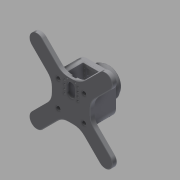
# Autodesk Inventor part: Arm - mounting v2
Saved by Autodesk Inventor 2017 (Build 210142000, 142)
## iProperties
Created: 2017-04-12
Part Number: Arm - mounting v2
Material: Generic
Document SubType Name: Modeling
Designer: Ali
Density: 1 g/cm^3
Appearance: Default
Author: Ali
Autodesk Inventor part; units mm, degrees
ref_plane "YZ Plane" through (0, 0, 0) normal (1, 0, 0) x (0, 1, 0)
ref_plane "XZ Plane" through (0, 0, 0) normal (0, 1, 0) x (-1, 0, 0)
ref_plane "XY Plane" through (0, 0, 0) normal (0, 0, 1) x (1, 0, 0)
sketch "Sketch1" plane through (0, 0, 0) normal (0, 1, 0) x (-1, 0, 0)
  line L0 (16.5, -22) -> (-16.5, -22) construction
  line L1 (-16.5, -22) -> (-16.5, 30.8666) construction
  line L2 (-16.5, 39) -> (16.5, 39)
  line L3 (16.5, 39) -> (16.5, 30.8666)
  line L4 (10.5, -16) -> (-10.5, -16) construction
  line L5 (-10.5, -16) -> (-10.5, 6.3097) construction
  line L6 (-10.5, 33) -> (10.5, 33)
  line L7 (10.5, 33) -> (10.5, 6.3097)
  arc A0 (-10.5, 6.3097) -> (10.5, 6.3097) centre (0, 0) ccw
  line L8 (0, 0) -> (0, -19.3758) construction
  arc A1 (16.5, 30.8666) -> (-16.5, 30.8666) centre (0, 0) ccw construction
  line L9 (16.5, 30.8666) -> (16.5, -22) construction
  line L10 (-16.5, 30.8666) -> (-16.5, 39)
  arc A2 (-16.5, 30.8666) -> (16.5, 30.8666) centre (0, 0) ccw
  line L11 (10.5, 6.3097) -> (10.5, -16) construction
  line L12 (-10.5, 6.3097) -> (-10.5, 33)
  arc A3 (10.5, 6.3097) -> (-10.5, 6.3097) centre (0, 0) ccw construction
  point P0 (0, -16)
  point P1 (0, -22)
  dimension "d0" = 21
  dimension "d1" = 24.5
  dimension "d2" = 6
  dimension "d3" = 33
  dimension "d4" = 6
  dimension "d5" = 16
  dimension "d6" = 6
  dimension "d7" = 70
  constraints: 26 end point, 10 parallel, 8 point on circle, 4 centre point, 4 perpendicular, 2 coincident, 2 horizontal, 2 midpoint, 2 point on line, 1 vertical
  measures "d0" distance of L6.start L6.end
  measures "d1" diameter of A0
  measures "d2" distance between parallel lines of L1 L5
  measures "d3" distance from line of point (0, 0) L6
  measures "d4" distance between parallel lines of L2 L6
  measures "d5" distance from line of point (0, 0) L4
  measures "d6" distance between parallel lines of L4 L0
  measures "d7" diameter of A1
extrude "Extrusion1" add sketch "Sketch1" along normal blind 3.5
sketch "Sketch2" plane through (0, 3.5, 0) normal (0, 1, 0) x (1, 0, 0)
  arc A0 (16.5, -30.8666) -> (-16.5, -30.8666) centre (0, 0) ccw projected
  line L0 (16.5, -39) -> (16.5, -30.8666) projected
  line L1 (-16.5, -39) -> (16.5, -39) projected
  line L2 (-16.5, -30.8666) -> (-16.5, -39) projected
  circle A1 centre (0, 0) radius 21
  dimension "d10" = 42
  constraints: 1 centre point, 1 coincident
  measures "d10" diameter of A1
extrude "Extrusion2" add sketch "Sketch2" along normal blind 8
sketch "Sketch3" plane through (0, 0, 0) normal (0, -1, 0) x (1, 0, 0)
  line L0 (-39, -39) -> (39, -39)
  line L1 (39, -39) -> (39, 39)
  line L2 (39, 39) -> (16.5, 39)
  line L3 (-39, 39) -> (-39, -39)
  line L4 (-39, -39) -> (39, 39) construction
  line L5 (39, -39) -> (-39, 39) construction
  line L6 (16.5, 39) -> (-16.5, 39) projected
  arc A0 (-16.5, 30.8666) -> (16.5, 30.8666) centre (0, 0) ccw projected
  line L7 (-16.5, 39) -> (-16.5, 30.8666) projected
  line L8 (-16.5, 39) -> (-39, 39)
  line L9 (16.5, 30.8666) -> (16.5, 39) projected
  line L10 (16.5, 39) -> (-16.5, 39)
  constraints: 18 end point, 4 parallel, 3 collinear, 2 midpoint, 2 perpendicular, 1 horizontal
extrude "Extrusion3" add sketch "Sketch3" against normal blind 8 contours L3 L8 L7 A0 L9 L2 L1 L0
sketch "Sketch4" plane through (0, 0, 0) normal (0, -1, 0) x (1, 0, 0)
  line L0 (-10.5, 6.3097) -> (-10.5, 33) projected
  line L1 (-10.5, 33) -> (10.5, 33) projected
  line L2 (10.5, 33) -> (10.5, 6.3097) projected
  arc A0 (10.5, 6.3097) -> (-10.5, 6.3097) centre (0, 0) ccw projected
  line L3 (-39, 39) -> (-39, -39) projected
  line L4 (-39, -39) -> (39, -39) projected
  line L5 (39, -39) -> (39, 39) projected
  line L6 (16, 39) -> (16, -12)
  line L7 (16, -12) -> (-16, -12)
  line L8 (-16, -12) -> (-16, 39)
  line L9 (0, 0) -> (0, 9.4966) construction
  line L10 (-16, 39) -> (-39, 39)
  line L11 (16, 39) -> (39, 39)
  point P0 (0, -12)
  dimension "d15" = 32
  dimension "d16" = 12
  constraints: 12 end point, 3 perpendicular, 1 centre point, 1 horizontal, 1 midpoint, 1 point on line, 1 vertical
  measures "d15" distance between parallel lines of L8 L6
  measures "d16" distance from line of point (0, 0) L7
extrude "Extrusion4" add sketch "Sketch4" along normal blind 32 contours L10 L8 L7 L6 L11 L5 L4 L3
fillet "Fillet1" radius 19.25 4 edges at (-39, -12, 39) (39, -12, 39) (39, -12, -39) (-39, -12, -39)
sketch "Sketch5" plane through (0, 8, 0) normal (0, 1, 0) x (1, 0, 0)
  arc A0 (-19.75, 39) -> (-39, 19.75) centre (-19.75, 19.75) ccw projected
  line L0 (-39, 19.75) -> (-39, -19.75) projected
  arc A1 (-39, -19.75) -> (-19.75, -39) centre (-19.75, -19.75) ccw projected
  line L1 (-19.75, -39) -> (-16.5, -39) projected
  line L2 (-16.5, -30.8666) -> (-16.5, -39) projected
  arc A2 (16.5, -30.8666) -> (-16.5, -30.8666) centre (0, 0) ccw projected
  line L3 (16.5, -39) -> (16.5, -30.8666) projected
  line L4 (16.5, -39) -> (19.75, -39) projected
  arc A3 (19.75, -39) -> (39, -19.75) centre (19.75, -19.75) ccw projected
  line L5 (39, -19.75) -> (39, 19.75) projected
  arc A4 (39, 19.75) -> (19.75, 39) centre (19.75, 19.75) ccw projected
  line L6 (19.75, 39) -> (-19.75, 39) projected
extrude "Extrusion5" add sketch "Sketch5" along normal up to surface (3.5 mm away)
sketch "Sketch6" plane through (0, -32, 0) normal (0, -1, 0) x (1, 0, 0)
  line L0 (-68.9878, -68.9878) -> (68.9878, 68.9878) construction
  line L1 (-58.3812, -79.5944) -> (-17.7868, -39)
  line L2 (58.3812, 79.5944) -> (17.7868, 39)
  arc A0 (-79.5944, -58.3812) -> (-58.3812, -79.5944) centre (-68.9878, -68.9878) ccw
  arc A1 (79.5944, 58.3812) -> (58.3812, 79.5944) centre (68.9878, 68.9878) ccw
  line L3 (0, 0) -> (195.1269, 0) construction
  line L4 (-68.9878, 68.9878) -> (68.9878, -68.9878) construction
  line L5 (-79.5944, 58.3812) -> (-39, 17.7868)
  line L6 (79.5944, -58.3812) -> (39, -17.7868)
  arc A2 (-58.3812, 79.5944) -> (-79.5944, 58.3812) centre (-68.9878, 68.9878) ccw
  arc A3 (58.3812, -79.5944) -> (79.5944, -58.3812) centre (68.9878, -68.9878) ccw
  line L7 (0, 0) -> (195.1269, 0) construction
  line L8 (-39, 39) -> (-17.7868, 39) construction
  line L9 (39, 39) -> (39, 17.7868) construction
  line L10 (39, -39) -> (17.7868, -39) construction
  line L11 (-39, -39) -> (-39, -17.7868) construction
  line L12 (-39, 39) -> (39, -39) construction
  line L13 (39, 39) -> (-39, -39) construction
  line L14 (39, -19.75) -> (39, 19.75) projected
  line L15 (-39, 17.7868) -> (17.7868, -39) construction
  line L16 (-17.7868, 39) -> (-58.3812, 79.5944)
  line L17 (17.7868, 39) -> (-39, -17.7868) construction
  line L18 (39, 17.7868) -> (79.5944, 58.3812)
  line L19 (39, -17.7868) -> (-17.7868, 39) construction
  line L20 (17.7868, -39) -> (58.3812, -79.5944)
  line L21 (-17.7868, -39) -> (39, 17.7868) construction
  line L22 (-39, -17.7868) -> (-79.5944, -58.3812)
  line L23 (-17.7868, -39) -> (-39, -39) construction
  line L24 (-39, -17.7868) -> (-39, 17.7868)
  line L25 (-39, 17.7868) -> (-39, 39) construction
  line L26 (-17.7868, 39) -> (17.7868, 39)
  line L27 (17.7868, 39) -> (39, 39) construction
  line L28 (39, 17.7868) -> (39, -17.7868)
  line L29 (39, -17.7868) -> (39, -39) construction
  line L30 (17.7868, -39) -> (-17.7868, -39)
  dimension "d22" = 45
  dimension "d23" = 30
  dimension "d24" = 45
  dimension "d25" = 30
  constraints: 64 end point, 36 parallel, 24 tangent, 9 perpendicular, 8 point on circle, 5 horizontal, 5 point on line, 4 centre point, 4 midpoint, 3 collinear, 3 equal length
  measures "d22" angle of L3 L0
  measures "d23" diameter of A1
  measures "d24" angle of L4 L7
  measures "d25" diameter of A3
extrude "Extrusion6" add sketch "Sketch6" along normal blind 8 separate body
fillet "Fillet2" radius 30 8 edges at (39, -36, 17.7868) (39, -36, -17.7868) (17.7868, -36, -39) (-17.7868, -36, -39) (-39, -36, -17.7868) (-39, -36, 17.7868) (-17.7868, -36, 39) (17.7868, -36, 39)
sketch "Sketch7" plane through (0, -32, 0) normal (0, 1, 0) x (1, 0, 0)
  line L0 (-10, -33) -> (10, -33)
  line L1 (-10, 6) -> (10, 6)
  line L2 (-10, -33) -> (-10, 6)
  line L3 (10, -33) -> (10, 6)
  line L4 (0, 0) -> (0, 4.84) construction
  line L5 (-4.5, -33) -> (4.5, -33)
  line L6 (4.5, -33) -> (4.5, -49)
  line L7 (4.5, -49) -> (-4.5, -49)
  line L8 (-4.5, -49) -> (-4.5, -33)
  point P0 (0, -33)
  point P1 (0, -49)
  dimension "d29" = 33
  dimension "d30" = 6
  dimension "d31" = 20
  dimension "d34" = 16
  dimension "d35" = 9
  constraints: 18 end point, 3 horizontal, 3 point on line, 3 vertical, 2 midpoint, 2 parallel, 1 perpendicular
  measures "d29" distance from line of L4.start L0
  measures "d30" distance from line of L1 L4.start
  measures "d31" distance between parallel lines of L3 L2
  measures "d34" distance between parallel lines of L0 L7
  measures "d35" distance between parallel lines of L6 L8
extrude "Extrusion7" cut sketch "Sketch7" against normal blind 3 bodies 2
sketch "Sketch8" plane through (0, -40, 0) normal (0, -1, 0) x (1, 0, 0)
  line L0 (4.5, 39) -> (-4.5, 39) construction
  line L1 (4.5, 33) -> (4.5, 39) construction
  line L2 (10, 33) -> (4.5, 33) construction
  line L3 (10, -6) -> (10, 33) construction
  line L4 (-10, -6) -> (10, -6) construction
  line L5 (-10, 33) -> (-10, -6) construction
  line L6 (-4.5, 33) -> (-10, 33) construction
  line L7 (-4.5, 39) -> (-4.5, 33) construction
  line L8 (0, 0) -> (0, 36)
  line L9 (-13.5, 36) -> (0, 36) construction
  line L10 (-13.5, 36) -> (-13.5, -8.0109) construction
  point P0 (-8, 36)
  point P1 (-13.5, 30.5)
  point P2 (-13.5, 22.5)
  point P3 (-13.5, 14.5)
  point P4 (-13.5, 6.5)
  point P5 (8, 36)
  point P6 (13.5, 30.5)
  point P7 (13.5, 22.5)
  point P8 (13.5, 14.5)
  point P9 (13.5, 6.5)
  dimension "d36" = 27
  dimension "d37" = 36
  dimension "d38" = 6.5
  dimension "d39" = 8
  dimension "d40" = 8
  dimension "d41" = 8
  dimension "d42" = 16
  constraints: 6 end point, 5 point on line, 5 symmetric about line, 2 vertical, 1 horizontal
  measures "d36" diameter of L10 L8
  measures "d37" distance from line of L8.start L9
  measures "d38" vertical distance of L8.start point (-13.5, 6.5)
  measures "d39" distance of point (-13.5, 14.5) point (-13.5, 6.5)
  measures "d40" distance of point (-13.5, 22.5) point (-13.5, 14.5)
  measures "d41" distance of point (-13.5, 30.5) point (-13.5, 22.5)
  measures "d42" diameter of point (-8, 36) L8
hole "Hole1" at (-8, -40, 36) at (-13.5, -40, 30.5) at (-13.5, -40, 22.5) at (-13.5, -40, 14.5) at (-13.5, -40, 6.5) at (13.5, -40, 30.5) at (8, -40, 36) at (13.5, -40, 22.5) at (13.5, -40, 14.5) at (13.5, -40, 6.5) direction (0, 1, 0) diameter 2 end through all counterbore diameter 4 counterbore depth 6 bodies 2
ref_plane "Work Plane1" through (0, 3.5, 0) normal (0, -1, 0) x (1, 0, 0)
split body "Split1" result two bodies by plane through (0, 3.5, 0) normal (0, -1, 0) bodies 1 first body at (-23.6667, -31.5, 15.5833)
sketch "Sketch9" plane through (0, 3.5, 0) normal (0, 1, 0) x (1, 0, 0)
  circle A0 centre (-13.5, -6.5) radius 1 projected
  circle A1 centre (-13.5, -14.5) radius 1 projected
  circle A2 centre (-13.5, -22.5) radius 1 projected
  circle A3 centre (-13.5, -30.5) radius 1 projected
  circle A4 centre (-8, -36) radius 1 projected
  circle A5 centre (8, -36) radius 1 projected
  circle A6 centre (13.5, -30.5) radius 1 projected
  circle A7 centre (13.5, -22.5) radius 1 projected
  circle A8 centre (13.5, -14.5) radius 1 projected
  circle A9 centre (13.5, -6.5) radius 1 projected
  point P0 (0, 0)
hole "Hole2" at (0, 3.5, 0) at (-8, 3.5, 36) at (8, 3.5, 36) at (13.5, 3.5, 30.5) at (13.5, 3.5, 22.5) at (13.5, 3.5, 14.5) at (13.5, 3.5, 6.5) at (-13.5, 3.5, 6.5) at (-13.5, 3.5, 14.5) at (-13.5, 3.5, 22.5) at (-13.5, 3.5, 30.5) direction (0, -1, 0) diameter 2 end through all counterbore diameter 4 counterbore depth 2 bodies 3
sketch "Sketch10" plane through (0, 3.5, 0) normal (0, 1, 0) x (1, 0, 0)
  line L0 (-26, -26) -> (26, -26)
  line L1 (26, -26) -> (26, 26)
  line L2 (26, 26) -> (-26, 26)
  line L3 (-26, 26) -> (-26, -26)
  line L4 (-26, -26) -> (26, 26) construction
  line L5 (26, -26) -> (-26, 26) construction
  point P0 (0, 0)
  point P1 (0, 0)
  point P2 (0, 0)
  dimension "d58" = 52
  dimension "d59" = 52
  constraints: 12 end point, 5 coincident, 3 midpoint, 2 parallel, 1 horizontal, 1 perpendicular
  measures "d58" distance of L1.end L2.end
  measures "d59" distance of L0.end L1.end
hole "Hole3" at (-26, 3.5, -26) at (26, 3.5, -26) at (26, 3.5, 26) at (-26, 3.5, 26) direction (0, -1, 0) diameter 12 end through all bodies 3
sketch "Sketch11" plane through (0, -32, 0) normal (0, 1, 0) x (1, 0, 0)
  circle A0 centre (-26, 26) radius 6 projected
  circle A1 centre (-26, -26) radius 6 projected
  circle A2 centre (26, -26) radius 6 projected
  circle A3 centre (26, 26) radius 6 projected
  point P0 (0, 0)
extrude "Extrusion8" add sketch "Sketch11" along normal up to surface (35.5 mm away) bodies 2
sketch "Sketch12" plane through (0, -40, 0) normal (0, -1, 0) x (1, 0, 0)
  circle A0 centre (-26, 26) radius 6 projected
  circle A1 centre (-26, -26) radius 6 projected
  circle A2 centre (26, -26) radius 6 projected
  circle A3 centre (26, 26) radius 6 projected
  point P0 (0, 0)
hole "Hole4" at (-26, -40, 26) at (-26, -40, -26) at (26, -40, -26) at (26, -40, 26) direction (0, 1, 0) diameter 4.2 end through all counterbore diameter 8 counterbore depth 4 bodies 2 4
sketch "Sketch13" plane through (0, 11.5, 0) normal (0, 1, 0) x (1, 0, 0)
  circle A0 centre (-26, 26) radius 2.1 projected
  circle A1 centre (-26, -26) radius 2.1 projected
  circle A2 centre (26, -26) radius 2.1 projected
  circle A3 centre (26, 26) radius 2.1 projected
  circle A4 centre (-26, 26) radius 2.1 projected
  line L0 (-21.9008, 26) -> (-23.9504, 22.45)
  line L1 (-23.9504, 22.45) -> (-28.0496, 22.45)
  line L2 (-28.0496, 22.45) -> (-30.0992, 26)
  line L3 (-30.0992, 26) -> (-28.0496, 29.55)
  line L4 (-28.0496, 29.55) -> (-23.9504, 29.55)
  line L5 (-23.9504, 29.55) -> (-21.9008, 26)
  line L6 (21.9008, 26) -> (23.9504, 29.55)
  line L7 (23.9504, 29.55) -> (28.0496, 29.55)
  line L8 (28.0496, 29.55) -> (30.0992, 26)
  line L9 (30.0992, 26) -> (28.0496, 22.45)
  line L10 (28.0496, 22.45) -> (23.9504, 22.45)
  line L11 (23.9504, 22.45) -> (21.9008, 26)
  line L12 (21.9008, -26) -> (23.9504, -22.45)
  line L13 (23.9504, -22.45) -> (28.0496, -22.45)
  line L14 (28.0496, -22.45) -> (30.0992, -26)
  line L15 (30.0992, -26) -> (28.0496, -29.55)
  line L16 (28.0496, -29.55) -> (23.9504, -29.55)
  line L17 (23.9504, -29.55) -> (21.9008, -26)
  line L18 (-21.9008, -26) -> (-23.9504, -29.55)
  line L19 (-23.9504, -29.55) -> (-28.0496, -29.55)
  line L20 (-28.0496, -29.55) -> (-30.0992, -26)
  line L21 (-30.0992, -26) -> (-28.0496, -22.45)
  line L22 (-28.0496, -22.45) -> (-23.9504, -22.45)
  line L23 (-23.9504, -22.45) -> (-21.9008, -26)
  point P0 (0, 0)
  dimension "d76" = 7.1
  dimension "d77" = 7.1
  constraints: 48 end point, 4 coincident, 2 collinear, 2 horizontal, 52 other
  measures "d76" distance between parallel lines of L4 L1
  measures "d77" distance between parallel lines of L22 L19
extrude "Extrusion9" cut sketch "Sketch13" against normal blind 5 bodies 4
sketch "Sketch14" plane through (0, 11.5, 0) normal (0, 1, 0) x (1, 0, 0)
  circle A0 centre (0, 0) radius 29.5
  circle A1 centre (0, 0) radius 21 projected
  dimension "d80" = 59
  constraints: 1 centre point, 1 coincident
  measures "d80" diameter of A0
extrude "Extrusion10" add sketch "Sketch14" along normal blind 17.5 bodies 4
sketch "Sketch15" plane through (0, 29, 0) normal (0, 1, 0) x (1, 0, 0)
  circle A0 centre (0, 0) radius 26
  circle A1 centre (0, 0) radius 21 projected
  point P0 (0, 0)
  dimension "d83" = 52
  constraints: 1 centre point, 1 coincident
  measures "d83" diameter of A0
extrude "Extrusion11" add sketch "Sketch15" along normal blind 7 bodies 4
sketch "Sketch16" plane through (0, 36, 0) normal (0, 1, 0) x (1, 0, 0)
  circle A0 centre (0, 0) radius 23.5
  point P0 (0, 0)
  dimension "d86" = 47
  constraints: 1 centre point, 1 coincident
  measures "d86" diameter of A0
extrude "Extrusion12" cut sketch "Sketch16" against normal blind 23 bodies 4
chamfer "Chamfer1" distance 1.5 angle 45 1 edges at (-26, 36, 0)
sketch "Sketch17" plane through (0, -40, 0) normal (0, -1, 0) x (1, 0, 0)
  line L0 (0, 0) -> (0, 55.0964)
  line L1 (0, 24) -> (0, 12) construction
  line L2 (-8, 24) -> (-8, 12)
  line L3 (8, 12) -> (8, 24)
  arc A0 (8, 24) -> (-8, 24) centre (0, 24) ccw
  arc A1 (-8, 12) -> (8, 12) centre (0, 12) ccw
  point P0 (0, 18)
  dimension "d92" = 16
  dimension "d93" = 12
  dimension "d94" = 12
  constraints: 10 end point, 4 point on circle, 4 tangent, 2 centre point, 2 point on line, 1 midpoint, 1 parallel, 1 vertical
  measures "d92" diameter of A1
  measures "d93" distance of L3.start L3.end
  measures "d94" distance of L0.start L1.end
extrude "Extrusion13" cut sketch "Sketch17" against normal through all bodies 2
equation "\"d59\" = d58"
equation "\"d77\" = d76"
